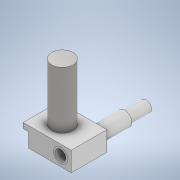
# Autodesk Inventor part: TuningPeg
Saved by Autodesk Inventor 2021 (Build 250183000, 183)
## iProperties
Created: 2021-02-02
Part Number: TuningPeg
Material: Generic
Document SubType Name: Modeling
Designer: garre
Density: 1 g/cm^3
Appearance: Default
Author: garre
Autodesk Inventor part; units mm, degrees
ref_plane "YZ Plane" through (0, 0, 0) normal (1, 0, 0) x (0, 1, 0)
ref_plane "XZ Plane" through (0, 0, 0) normal (0, 1, 0) x (-1, 0, 0)
ref_plane "XY Plane" through (0, 0, 0) normal (0, 0, 1) x (1, 0, 0)
sketch "Sketch1" plane through (0, 0, 0) normal (0, 1, 0) x (-1, 0, 0)
  circle A0 centre (0, 0) radius 4.7625
  line L0 (0, 0) -> (-11.9062, 0)
  line L1 (-11.9062, 0) -> (-11.9063, 7.9375)
  line L2 (-11.9063, 7.9375) -> (7.1437, 7.9375)
  line L3 (7.1437, 7.9375) -> (7.1437, -7.9375)
  line L4 (7.1437, -7.9375) -> (-11.9062, -7.9375)
  line L5 (-11.9062, -7.9375) -> (-11.9063, 7.9375)
  line L6 (0, -7.9375) -> (9.525, -7.9375)
  line L7 (9.525, -7.9375) -> (9.525, 7.9375)
  line L8 (9.525, 7.9375) -> (0, 7.9375)
  line L9 (0, 7.9375) -> (0, -7.9375)
  point P0 (-11.9063, 0)
  dimension "d0" = 9.525
  dimension "d9" = 15.875
  dimension "d10" = 7.9375
  dimension "d11" = 11.9062
  dimension "d12" = 7.1437
  dimension "d22" = 9.525
  constraints: 20 end point, 4 parallel, 3 horizontal, 2 perpendicular, 1 centre point, 1 coincident, 1 midpoint, 1 point on line, 1 vertical
  measures "d0" diameter of A0
  measures "d9" distance of L4.end L1.end
  measures "d10" distance of L0.end L1.end
  measures "d11" distance from line of L5 point (0, 0)
  measures "d12" distance from line of L3 point (0, 0)
  measures "d22" distance of L6.start L6.end
extrude "Extrusion1" add sketch "Sketch1" along normal blind 34.1313 contours A0 L9 | L9 L0 A0 | A0 L0 L9
extrude "Extrusion3" add sketch "Sketch1" along normal blind 8.7313 separate body contours A0 L9 L2 L3 L4 | A0 L0 L1 L2 L9 | L9 L4 L5 L0 A0
sketch "Sketch3" plane through (-7.1437, 0, 7.9375) normal (0, 0, 1) x (1, 0, 0)
  line L0 (0, 0) -> (0, 8.7313) projected
  line L1 (0, 4.3656) -> (19.05, 4.3656)
  line L2 (19.05, 0) -> (19.05, 8.7313) projected
  circle A0 centre (14.2875, 4.3656) radius 3.175
  circle A1 centre (14.2875, 4.3656) radius 2.3813
  point P0 (7.1437, 0)
  dimension "d15" = 6.35
  dimension "d16" = 4.7625
  dimension "d17" = 4.7625
  constraints: 2 centre point, 2 end point, 2 midpoint, 1 coincident, 1 point on line
  measures "d15" diameter of A0
  measures "d16" diameter of A1
  measures "d17" distance from line of L2 A0.centre
extrude "Extrusion4" add sketch "Sketch3" against normal blind 28.575 separate body contours A1 L1 A0 | L1 A0 A1
extrude "Extrusion5" cut sketch "Sketch3" against normal up to surface (15.875 mm away) contours A1 L1 | L1 A1 bodies 2
sketch "Sketch4" plane through (0, 8.7313, 0) normal (0, 1, 0) x (1, 0, 0)
  line L0 (-7.1437, -7.9375) -> (11.9063, -7.9375) projected
  line L1 (0, -7.9375) -> (-9.525, -7.9375)
  line L2 (11.9062, 7.9375) -> (-7.1437, 7.9375) projected
  line L3 (0, 7.9375) -> (-9.525, 7.9375)
  line L4 (-9.525, 7.9375) -> (-9.525, -7.9375)
  line L5 (-7.1437, 7.9375) -> (-7.1437, -7.9375) projected
  line L6 (-7.1437, -7.9375) -> (-7.1437, 7.9375)
  line L7 (0, 0) -> (0, -7.9375)
  point P0 (-7.1437, -7.9375)
  point P1 (-7.1437, 7.9375)
  dimension "d23" = 9.525
  constraints: 10 end point, 2 collinear, 2 perpendicular, 2 point on line, 1 horizontal
  measures "d23" distance of L1.start L1.end
extrude "Extrusion6" add sketch "Sketch4" against normal blind 2.3813 bodies 2
sketch "Sketch5" plane through (-7.1437, 0, 7.9375) normal (0, 0, 1) x (1, 0, 0)
  line L0 (19.05, 8.7313) -> (-2.3813, 8.7313) projected
  line L1 (7.1437, 8.7313) -> (7.1437, 34.1313)
  line L2 (11.9062, 34.1313) -> (2.3813, 34.1313) projected
  circle A0 centre (7.1437, 30.9563) radius 1.5875
  point P0 (7.1437, 0)
  dimension "d26" = 3.175
  dimension "d27" = 3.175
  constraints: 2 end point, 2 point on line, 1 centre point, 1 midpoint
  measures "d26" distance from line of L2 A0.centre
  measures "d27" diameter of A0
sketch "Sketch6" plane through (7.1438, 4.3656, -20.6375) normal (0, 0, -1) x (-1, 0, 0)
  circle A0 centre (0, 0) radius 2.3721
  point P0 (7.1438, -4.3656)
  constraints: 1 centre point
extrude "Extrusion7" add sketch "Sketch6" along normal blind 9.525 bodies 3
equation "\"d0\" = tuningPegDiameter"
equation "\"d9\" = 2 * lockOffset"
equation "\"d10\" = lockOffset"
equation "\"d11\" = lockLongYOffset"
equation "\"d12\" = lockShortYOffset"
equation "\"d22\" = mountExtension"
equation "\"d1\" = tuningPegDepth"
equation "\"d13\" = lockWidth"
equation "\"d15\" = screwOutsideDiameter"
equation "\"d16\" = screwInsideDiameter"
equation "\"d17\" = screwOffset"
equation "\"d20\" = screwExtension"
equation "\"d23\" = mountExtension"
equation "\"d24\" = mountPlateDepth"
equation "\"tuningPegDiameter\" = 9.525"
equation "\"screwOffset\" = 4.7625"
equation "\"screwOutsideDiameter\" = 6.35"
equation "\"screwInsideDiameter\" = 4.7625"
equation "\"screwExtension\" = 12.7"
equation "\"mountPlateDepth\" = 2.38125"
equation "\"holeOffset\" = 3.175"
equation "\"lockOffset\" = 7.9375"
equation "\"mountExtension\" = 9.525"
equation "\"tuningPegDepth\" = 34.13125"
equation "\"lockWidth\" = 8.73125"
equation "\"lockLongYOffset\" = 11.90625"
equation "\"lockShortYOffset\" = 7.14375"
body "Solid1"
body "Solid2"
body "Solid3"
